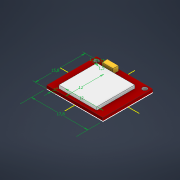
# Autodesk Inventor part: GSMModul
Saved by Autodesk Inventor 2021 (Build 250183000, 183)
## iProperties
Created: 2020-12-16
Part Number: GSMModul
Material: Generisch
Document SubType Name: Modeling
Designer: laure
Density: 1 g/cm^3
Appearance: Vorgabe
Author: laure
Autodesk Inventor part; units mm, degrees
ref_plane "YZ Plane" through (0, 0, 0) normal (1, 0, 0) x (0, 1, 0)
ref_plane "XZ Plane" through (0, 0, 0) normal (0, 1, 0) x (-1, 0, 0)
ref_plane "XY Plane" through (0, 0, 0) normal (0, 0, 1) x (1, 0, 0)
sketch "Skizze1" plane through (0, 0, 0) normal (0, 1, 0) x (-1, 0, 0)
  line L0 (8.9, -7.9) -> (-8.9, -7.9)
  line L1 (-8.9, -7.9) -> (-8.9, 7.9)
  line L2 (-8.9, 7.9) -> (8.9, 7.9)
  line L3 (8.9, 7.9) -> (8.9, -7.9)
  line L4 (12.46, 0) -> (-12.46, 0) projected
  line L5 (0, -11.06) -> (0, 11.06) projected
  line L6 (6, -5.1) -> (-6, -5.1)
  line L7 (-6, -5.1) -> (-6, 6.9)
  line L8 (-6, 6.9) -> (6, 6.9)
  line L9 (6, 6.9) -> (6, -5.1)
  circle A0 centre (7.65, -6.65) radius 0.75
  circle A1 centre (-7.65, -6.65) radius 0.75
  dimension "d0" = 17.8
  dimension "d1" = 15.8
  dimension "d3" = 12
  dimension "d4" = 12
  dimension "d5" = 1
  dimension "d15" = 1.5
  dimension "d16" = 1.25
  dimension "d17" = 1.25
  constraints: 16 end point, 4 parallel, 2 centre point, 2 horizontal, 2 perpendicular, 1 symmetric about line, 4 other
  measures "d0" distance of L1.end L2.end
  measures "d1" distance between parallel lines of L2 L0
  measures "d3" distance between parallel lines of L7 L9
  measures "d4" distance between parallel lines of L8 L6
  measures "d5" distance between parallel lines of L8 L2
  measures "d15" diameter of A0
  measures "d16" distance from line of L0 A0.centre
  measures "d17" distance from line of L3 A0.centre
extrude "Extrusion1" add sketch "Skizze1" along normal blind 1 contours L0 L5 L6 L9 L4 L3 | L0 L1 L4 L7 L6 L5 | L4 L9 L8 L5 L2 L3 | L6 L7 L4 L5 | L5 L4 L9 L6 | L4 L5 L8 L9 | L1 L2 L5 L8 L7 L4 | L4 L7 L8 L5 | A0 | A1
extrude "Extrusion2" add sketch "Skizze1" along normal blind 2 contours L6 L7 L4 L5 | L5 L4 L9 L6 | L4 L5 L8 L9 | L4 L7 L8 L5
sketch "Skizze2" plane through (0, 1, 0) normal (0, 1, 0) x (1, 0, 0)
  line L0 (-4.8872, 7.3) -> (-1.3872, 7.3)
  line L1 (-1.3872, 7.3) -> (-1.3872, 5.6)
  line L2 (-1.3872, 5.6) -> (-4.8872, 5.6)
  line L3 (-4.8872, 5.6) -> (-4.8872, 7.3)
  line L4 (6, 5.1) -> (-6, 5.1) projected
  point P0 (0, 0)
  dimension "d10" = 3.5
  dimension "d11" = 1.7
  dimension "d12" = 0.5
  constraints: 8 end point, 2 parallel, 1 horizontal, 1 perpendicular
  measures "d10" distance of L1.end L2.end
  measures "d11" distance between parallel lines of L2 L0
  measures "d12" distance between parallel lines of L4 L2
extrude "Extrusion3" add sketch "Skizze2" along normal blind 1.5
extrude "Extrusion4" cut sketch "Skizze1" along normal blind 1 contours A0 | A1
